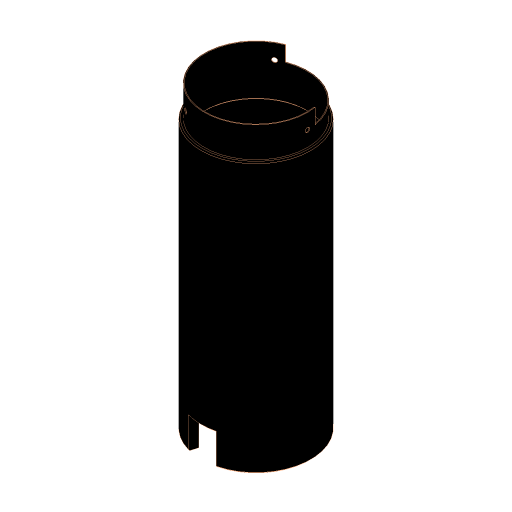
# Autodesk Inventor part: Lower skin
Saved by Autodesk Inventor 2024 (Build 280153000, 153)
## iProperties
Created: 2023-12-30
Part Number: Lower skin
Material: Plastic, Opaque White
Document SubType Name: Modeling
Designer: Jamie
Density: 0.952 g/cm^3
Appearance: Smooth - Light Orange
Author: Jamie
Autodesk Inventor part; units mm, degrees
ref_plane "XZ Plane" through (0, 0, 0) normal (0, 1, 0) x (-1, 0, 0)
ref_plane "XY Plane" through (0, 0, 0) normal (0, 0, 1) x (1, 0, 0)
sketch "Sketch1" plane through (0, 0, 0) normal (0, 1, 0) x (-1, 0, 0)
  circle A0 centre (0, 0) radius 36.1
  circle A1 centre (0, 0) radius 34.5
  dimension "d0" = 72.2
  dimension "d1" = 69
  constraints: 2 centre point, 2 coincident
  measures "d0" diameter of A0
  measures "d1" diameter of A1
extrude "Extrusion1" add sketch "Sketch1" along normal blind 178
ref_plane "Work Plane2" through (35, 0, 0) normal (1, 0, 0) x (0, 1, 0)
sketch "Sketch5" plane through (0, 178, 0) normal (0, 1, 0) x (1, 0, 0)
  circle A0 centre (0, 0) radius 34
  circle A1 centre (0, 0) radius 33.5
  dimension "d44" = 68
  dimension "d45" = 67
  constraints: 2 centre point, 2 coincident
  measures "d44" diameter of A0
  measures "d45" diameter of A1
extrude "Extrusion3" add sketch "Sketch5" along normal blind 20
sketch "Sketch6" plane through (0, 178, 0) normal (0, -1, 0) x (1, 0, 0)
  circle A0 centre (0, 0) radius 33.5
  circle A1 centre (0, 0) radius 34.5 projected
  circle A2 centre (0, 0) radius 35
  constraints: 2 centre point, 2 coincident
extrude "Extrusion4" add sketch "Sketch6" along normal blind 12.5 contours A1
ref_plane "Work Plane4" through (34, 0, 0) normal (1, 0, 0) x (0, 1, 0)
sketch "Sketch8" plane through (34, 0, 0) normal (1, 0, 0) x (0, 1, 0)
  line L0 (198, -34) -> (198, 34) projected
  point P0 (0, 0)
  point P1 (188, 0)
  dimension "d61" = 10
  measures "d61" distance from line of L0 point (188, 0)
hole "Hole4" at (34, 188, 0) direction (-1, 0, 0) diameter 3 depth 8 tip angle 118
pattern_circular "Circular Pattern2" count 3 over 360 about axis through (0, 0, 0) along (0, 1, 0) of "Hole4"
sketch "Sketch9" plane through (0, 0, 0) normal (0, -1, 0) x (1, 0, 0)
  line L0 (34.0588, 0) -> (34.0588, -5.5) construction
  circle A0 centre (0, 0) radius 34.5 projected
  circle A1 centre (0, 0) radius 33.5 projected
  arc A2 (33.4533, -8.4336) -> (34.0588, -5.5) centre (0, 0) ccw
  line L1 (34.0588, -5.5) -> (30, -5.5)
  line L2 (33.4533, -8.4336) -> (29.5747, -7.4557)
  arc A3 (29.5747, -7.4557) -> (30, -5.5) centre (0, 0) ccw
  line L3 (0, 0) -> (29.5747, -7.4557) construction
  line L4 (32.4837, -8.1891) -> (33.4533, -8.4336) construction
  point P0 (33.0454, -5.5)
  dimension "d72" = 5.5
  dimension "d73" = 0
  dimension "d82" = 4
  dimension "d83" = 30.5
  constraints: 11 end point, 8 point on circle, 2 centre point, 2 coincident, 1 horizontal, 1 vertical
  measures "d72" distance of L0.start L0.end
  measures "d73" vertical distance of point (0, 0) L0.start
  measures "d82" distance of L2.start L2.end
  measures "d83" radius of A3
extrude "Extrusion5" add sketch "Sketch9" against normal blind 100 contours L2 A1 L1 A0 | L2 A3 L1 A1 picked at (33.2774, -7.7311) picked at (31.6366, -7.4314)
mirror "Mirror1" about plane through (0, 0, 0) normal (0, 0, 1) of "Extrusion5"
pattern_circular "Circular Pattern3" count 3 over 360 about axis through (0, 0, 0) along (0, 1, 0) of "Extrusion5", "Mirror1"
chamfer "Chamfer1" distance 4 angle 45 6 edges at (-9.2887, 100, -29.0512) (-20.5147, 100, -22.5698) (-9.2887, 100, 29.0512) (-20.5147, 100, 22.5698) (29.8034, 100, 6.4814) (29.8034, 100, -6.4814)
sketch "Sketch10" plane through (0, 0, 0) normal (0, -1, 0) x (1, 0, 0)
  arc A0 (10.7588, 42.6767) -> (-12.021, 42.3385) centre (0, 0) ccw
  line L0 (0, 0) -> (10.7588, 42.6767) construction
  line L1 (0, 0) -> (-12.021, 42.3385) construction
  line L2 (10.7588, 42.6767) -> (0, 0)
  line L3 (-12.021, 42.3385) -> (0, 0)
  dimension "d88" = 30
  constraints: 8 end point, 2 collinear, 2 point on circle, 1 centre point
  measures "d88" angle of L0 L1
extrude "Extrusion6" cut sketch "Sketch10" against normal blind 20
mirror "Mirror2" about plane through (0, 0, 0) normal (0, 0, 1) of "Extrusion6"
chamfer "Chamfer2" distance 0.8 angle 45 4 edges at (36.1, 0, 0) (-28.8024, 0, -21.7631) (-28.8024, 0, 21.7631) (36.1, 178, 0)
chamfer "Chamfer3" distance 0.8 angle 45 2 edges at (-0.5359, 20, -36.096) (-0.5359, 20, 36.096)
sketch "Sketch11" plane through (0, 198, 0) normal (0, 1, 0) x (1, 0, 0)
  line L0 (0, 0) -> (-13.9367, 36.5912)
  line L1 (-8.3305, 29.3403) -> (-9.423, 33.1882) projected
  line L2 (0, 0) -> (48.0307, 7.7357)
  arc A0 (48.0307, 7.7357) -> (-13.9367, 36.5912) centre (12.7743, 12.9877) ccw
  line L3 (33.4533, 8.4336) -> (29.5747, 7.4557) projected
  dimension "d97" = 5
  dimension "d98" = 5
  constraints: 4 end point, 2 point on circle, 1 centre point
  measures "d97" angle of L1 L0
  measures "d98" angle of L3 L2
extrude "Extrusion7" cut sketch "Sketch11" against normal blind 10
chamfer "Chamfer4" distance 1 angle 45 1 edges at (34.5, 165.5, 0)
body "Solid1"
